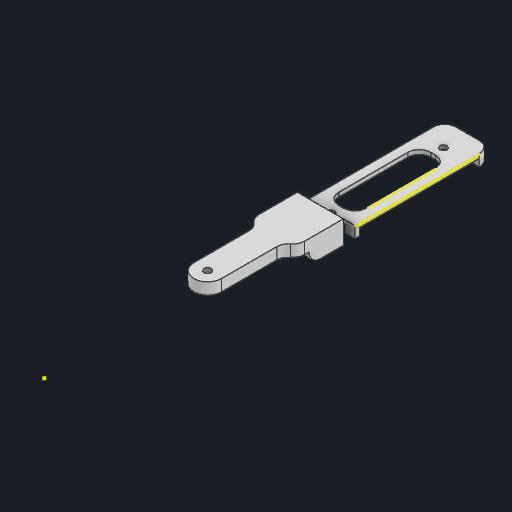
# Autodesk Inventor part: SideSensor
Saved by Autodesk Inventor 2022 (Build 260153000, 153)
## iProperties
Created: 2021-10-25
Part Number: SideSensor
Material: 一般
Document SubType Name: Modeling
Designer: shiok
Density: 1 g/cm^3
Appearance: 既定
Author: shiok
Autodesk Inventor part; units mm, degrees
ref_plane "YZ Plane" through (0, 0, 0) normal (1, 0, 0) x (0, 1, 0)
ref_plane "XZ Plane" through (0, 0, 0) normal (0, 1, 0) x (-1, 0, 0)
ref_plane "XY Plane" through (0, 0, 0) normal (0, 0, 1) x (1, 0, 0)
sketch "スケッチ1" plane through (0, 0, 0) normal (0, 1, 0) x (-1, 0, 0)
  line L0 (3, -32.5) -> (-3, -32.5)
  line L1 (-3, -32.5) -> (-3, -89.5)
  line L2 (3, -89.5) -> (3, -32.5)
  line L3 (-3, -89.5) -> (0, -89.5)
  line L4 (0, -89.5) -> (3, -89.5)
  point P0 (0, 0)
  point P1 (0, -35)
  point P2 (0, -40)
  point P3 (0, -50)
  dimension "d1" = 32.5
  dimension "d2" = 2.5
  dimension "d3" = 5
  dimension "d4" = 10
  dimension "d5" = 6
  dimension "d6" = 89.5
  constraints: 10 end point, 4 vertical alignment, 2 collinear, 2 horizontal, 1 parallel, 1 perpendicular
  measures "d1" distance from line of L0 point (0, 0)
  measures "d2" distance from line of L0 point (0, -35)
  measures "d3" distance of point (0, -40) point (0, -35)
  measures "d4" distance of point (0, -50) point (0, -40)
  measures "d5" distance of L0.start L0.end
  measures "d6" distance from line of point (0, 0) L4
extrude "押し出し1" add sketch "スケッチ1" along normal blind 2.5
sketch "スケッチ2" plane through (0, 2.5, 0) normal (0, 1, 0) x (1, 0, 0)
  line L0 (-3, 32.5) -> (3, 32.5) projected
  line L1 (0, 32.5) -> (0, 35) construction
  point P0 (0, 0)
  point P1 (0, 40)
  point P2 (0, 50)
  dimension "d9" = 2.5
  dimension "d10" = 5
  dimension "d11" = 10
  constraints: 2 end point, 2 vertical alignment, 1 midpoint, 1 vertical
  measures "d9" distance from line of L0 L1.end
  measures "d10" distance of point (0, 40) L1.end
  measures "d11" distance of point (0, 50) point (0, 40)
hole "穴1" at (0, 2.5, -50) at (0, 2.5, -40) at (0, 2.5, -35) direction (0, -1, 0) diameter 1.567 depth 2.5 thread size "M2x0.4" class "6H" standard "ISO Metric profile"
sketch "スケッチ3" plane through (0, 2.5, 0) normal (0, 1, 0) x (1, 0, 0)
  line L0 (-5, 50) -> (-5, 89.5)
  line L1 (-5, 89.5) -> (5, 89.5)
  line L2 (5, 89.5) -> (5, 50)
  circle A0 centre (0, 50) radius 0.7835 projected
  line L3 (3, 89.5) -> (-3, 89.5) projected
  line L4 (5, 50) -> (0, 50)
  line L5 (0, 50) -> (-5, 50)
  point P0 (0, 0)
  point P1 (0.5, 89.5)
  point P2 (-0.5, 89.5)
  point P3 (-0.7835, 50)
  point P4 (0.7835, 50)
  dimension "d22" = 10
  constraints: 10 end point, 2 collinear, 2 equal length, 1 horizontal, 1 vertical
  measures "d22" distance between parallel lines of L2 L0
extrude "押し出し2" add sketch "スケッチ3" against normal up to surface (2.5 mm away) contours L0 L1 L2 L4 A0 L5
fillet "フィレット3" radius 2.5 6 edges at (5, 1.25, -50) (3, 1.25, -50) (-5, 1.25, -50) (-3, 1.25, -50) (5, 1.25, -89.5) (-5, 1.25, -89.5)
sketch "スケッチ4" plane through (0, 0, 0) normal (0, -1, 0) x (1, 0, 0)
  line L0 (-2.5, -89.5) -> (2.5, -89.5) projected
  line L1 (2.5, -89.5) -> (-2.5, -89.5) construction
  line L2 (0, -89.5) -> (0, -86.75) construction
  line L3 (0, -86.75) -> (0, -62.25) construction
  circle A0 centre (0, -50) radius 0.7835 projected
  point P0 (0, 0)
  point P1 (0, -74.5)
  dimension "d36" = 12.25
  dimension "d42" = 24.5
  constraints: 4 end point, 2 coincident, 2 midpoint, 1 point on line, 1 vertical
  measures "d36" distance of L3.end A0.centre
  measures "d42" distance of point (0, -86.75) point (0, -62.25)
hole "穴2" at (0, 0, -86.75) at (0, 0, -62.25) direction (0, 1, 0) diameter 1.567 depth 2.5 thread size "M2x0.4" class "6H" standard "ISO Metric profile"
sketch "スケッチ5" plane through (0, 0, 0) normal (0, -1, 0) x (1, 0, 0)
  line L0 (-2.5, -89.5) -> (2.5, -89.5) projected
  line L1 (2.5, -89.5) -> (-2.5, -89.5) construction
  line L2 (0.5, -64.5) -> (-0.5, -64.5)
  line L3 (-3, -67) -> (-3, -82)
  line L4 (-0.5, -84.5) -> (0.5, -84.5)
  line L5 (3, -82) -> (3, -67)
  line L6 (3, -64.5) -> (-3, -84.5) construction
  line L7 (3, -84.5) -> (-3, -64.5) construction
  circle A0 centre (0, -62.25) radius 0.7835 construction
  circle A1 centre (0, -86.75) radius 0.7835 construction
  line L8 (0, -62.25) -> (0, -86.75) construction
  arc A2 (3, -67) -> (0.5, -64.5) centre (0.5, -67) ccw
  arc A3 (0.5, -84.5) -> (3, -82) centre (0.5, -82) ccw
  arc A4 (-3, -82) -> (-0.5, -84.5) centre (-0.5, -82) ccw
  arc A5 (-0.5, -64.5) -> (-3, -67) centre (-0.5, -67) ccw
  point P0 (0, 0)
  point P1 (0, -74.5)
  dimension "d37" = 20
  dimension "d38" = 6
  dimension "d39" = 2.5
  constraints: 14 end point, 8 point on circle, 8 point on line, 8 tangent, 4 centre point, 3 equal radius, 3 midpoint, 2 parallel, 1 horizontal, 1 perpendicular, 1 vertical
  measures "d37" distance of L7.end L6.end
  measures "d38" distance of L6.end L7.start
  measures "d39" radius of A2
extrude "押し出し3" cut sketch "スケッチ5" against normal up to surface (2.5 mm away)
sketch "スケッチ6" plane through (0, 2.5, 0) normal (0, 1, 0) x (1, 0, 0)
  circle A0 centre (0, 40) radius 0.7835 projected
  circle A1 centre (0, 35) radius 0.7835 projected
  point P0 (0, 0)
extrude "押し出し4" add sketch "スケッチ6" against normal up to surface (2.5 mm away)
fillet "フィレット4" radius 3 2 edges at (3, 1.25, -32.5) (-3, 1.25, -32.5)
sketch "スケッチ8" plane through (0, 2.5, 0) normal (0, 1, 0) x (1, 0, 0)
  circle A0 centre (0, 50) radius 0.7835 projected
  point P0 (0, 0)
extrude "押し出し5" add sketch "スケッチ8" against normal up to surface (2.5 mm away)
sketch "スケッチ9" plane through (0, 0, 0) normal (0, -1, 0) x (1, 0, 0)
  arc A0 (3, -35.5) -> (-3, -35.5) centre (0, -35.5) ccw projected
  line L0 (-3, -47.5505) -> (-3, -35.5) projected
  arc A1 (-4, -49.5505) -> (-3, -47.5505) centre (-5.5, -47.5505) ccw projected
  arc A2 (-4, -49.5505) -> (-5, -51.5505) centre (-2.5, -51.5505) ccw projected
  line L1 (-5, -51.5505) -> (-5, -87) projected
  arc A3 (-5, -87) -> (-2.5, -89.5) centre (-2.5, -87) ccw projected
  line L2 (-2.5, -89.5) -> (2.5, -89.5) projected
  arc A4 (2.5, -89.5) -> (5, -87) centre (2.5, -87) ccw projected
  line L3 (5, -87) -> (5, -51.5505) projected
  arc A5 (5, -51.5505) -> (4, -49.5505) centre (2.5, -51.5505) ccw projected
  arc A6 (3, -47.5505) -> (4, -49.5505) centre (5.5, -47.5505) ccw projected
  line L4 (3, -35.5) -> (3, -47.5505) projected
  line L5 (3, -67) -> (3, -82) projected
  arc A7 (0.5, -84.5) -> (3, -82) centre (0.5, -82) ccw projected
  line L6 (0.5, -84.5) -> (-0.5, -84.5) projected
  arc A8 (-3, -82) -> (-0.5, -84.5) centre (-0.5, -82) ccw projected
  line L7 (-3, -82) -> (-3, -67) projected
  arc A9 (-0.5, -64.5) -> (-3, -67) centre (-0.5, -67) ccw projected
  line L8 (-0.5, -64.5) -> (0.5, -64.5) projected
  arc A10 (3, -67) -> (0.5, -64.5) centre (0.5, -67) ccw projected
  circle A11 centre (0, -86.75) radius 0.7835 projected
  circle A12 centre (0, -62.25) radius 0.7835 projected
  line L9 (-5, -51.5505) -> (-5, -87) projected
  line L10 (5, -89.5) -> (-5, -89.5)
  line L11 (-5, -89.5) -> (-5, -59.5)
  line L12 (-5, -59.5) -> (5, -59.5)
  line L13 (5, -59.5) -> (5, -89.5)
  line L14 (5, -87) -> (5, -51.5505) projected
  line L15 (-2.5, -89.5) -> (2.5, -89.5) projected
  line L16 (5, -59.5) -> (3, -59.5)
  line L17 (3, -59.5) -> (3, -63.5)
  line L18 (3, -63.5) -> (5, -63.5)
  line L19 (5, -63.5) -> (5, -59.5)
  line L20 (0, -35.5) -> (0, -86.75)
  line L21 (-3, -59.5) -> (-3, -63.5)
  line L22 (-3, -63.5) -> (-5, -63.5)
  point P0 (0, 0)
  dimension "d56" = 30
  dimension "d67" = 2
  dimension "d68" = 4
  constraints: 22 end point, 4 parallel, 3 symmetric about line, 2 collinear, 2 horizontal, 2 perpendicular, 1 point on line, 1 vertical
  measures "d56" distance of L10.end L11.end
  measures "d67" distance of L18.end L17.end
  measures "d68" distance of L17.end L16.end
extrude "押し出し6" cut sketch "スケッチ9" against normal blind 1.6 contours L3 A4 L2 A3 L1 L22 L21 L12 L17 L18
sketch "スケッチ10" plane through (0, 2.5, 0) normal (0, 1, 0) x (1, 0, 0)
  arc A0 (-2.5, 89.5) -> (-5, 87) centre (-2.5, 87) ccw projected
  line L0 (-5, 87) -> (5, 87)
  line L1 (5, 87) -> (5, 92)
  line L2 (5, 92) -> (-5, 92)
  line L3 (-5, 92) -> (-5, 87)
  circle A1 centre (0, 86.75) radius 0.7835 projected
  point P0 (0, 0)
  point P1 (-0.7425, 87)
  point P2 (0.7425, 87)
  dimension "d59" = 10
  dimension "d60" = 5
  constraints: 8 end point, 2 parallel, 1 horizontal, 1 perpendicular
  measures "d59" distance of L2.end L1.end
  measures "d60" distance of L1.end L0.end
extrude "押し出し7" add sketch "スケッチ10" against normal up to surface (0.9 mm away) contours L3 L2 L1 L0 A1
sketch "スケッチ11" plane through (0, 1.6, 0) normal (0, -1, 0) x (1, 0, 0)
  line L0 (5, -63.5) -> (5, -92) projected
  line L1 (-5, -92) -> (-5, -51.5505) projected
  line L2 (5, -89.5) -> (-5, -89.5)
  line L3 (-5, -89.5) -> (-5, -92)
  line L4 (-5, -92) -> (5, -92)
  line L5 (5, -92) -> (5, -89.5)
  line L6 (5, -92) -> (-5, -92) projected
  point P0 (0, 0)
  point P1 (5, -59.5)
  dimension "d63" = 2.5
  constraints: 8 end point, 2 parallel, 2 point on line, 1 collinear, 1 horizontal, 1 perpendicular
  measures "d63" distance between parallel lines of L4 L2
extrude "押し出し8" add sketch "スケッチ11" along normal up to surface (1.6 mm away)
fillet "フィレット5" radius 2.5 2 edges at (5, 1.25, -92) (-5, 1.25, -92)
sketch "スケッチ12" plane through (0, 2.5, 0) normal (0, 1, 0) x (1, 0, 0)
  line L0 (5, 32.5) -> (-5, 32.5)
  line L1 (-5, 32.5) -> (-5, 57.5)
  line L2 (-5, 57.5) -> (5, 57.5)
  line L3 (5, 57.5) -> (5, 32.5)
  line L4 (5, 51.5505) -> (5, 89.5) projected
  arc A0 (-3, 35.5) -> (3, 35.5) centre (0, 35.5) ccw projected
  arc A1 (-2.5, 92) -> (-5, 89.5) centre (-2.5, 89.5) ccw projected
  line L5 (-5, 89.5) -> (-5, 51.5505) projected
  arc A2 (-5, 51.5505) -> (-4, 49.5505) centre (-2.5, 51.5505) ccw projected
  arc A3 (-3, 47.5505) -> (-4, 49.5505) centre (-5.5, 47.5505) ccw projected
  line L6 (-3, 47.5505) -> (-3, 35.5) projected
  arc A4 (-3, 35.5) -> (3, 35.5) centre (0, 35.5) ccw projected
  line L7 (3, 35.5) -> (3, 47.5505) projected
  arc A5 (4, 49.5505) -> (3, 47.5505) centre (5.5, 47.5505) ccw projected
  arc A6 (4, 49.5505) -> (5, 51.5505) centre (2.5, 51.5505) ccw projected
  line L8 (5, 51.5505) -> (5, 89.5) projected
  arc A7 (5, 89.5) -> (2.5, 92) centre (2.5, 89.5) ccw projected
  line L9 (2.5, 92) -> (-2.5, 92) projected
  circle A8 centre (0, 86.75) radius 0.7835 projected
  circle A9 centre (0, 62.25) radius 0.7835 projected
  line L10 (3, 82) -> (3, 67) projected
  arc A10 (0.5, 64.5) -> (3, 67) centre (0.5, 67) ccw projected
  line L11 (0.5, 64.5) -> (-0.5, 64.5) projected
  arc A11 (-3, 67) -> (-0.5, 64.5) centre (-0.5, 67) ccw projected
  line L12 (-3, 67) -> (-3, 82) projected
  arc A12 (-0.5, 84.5) -> (-3, 82) centre (-0.5, 82) ccw projected
  line L13 (-0.5, 84.5) -> (0.5, 84.5) projected
  arc A13 (3, 82) -> (0.5, 84.5) centre (0.5, 82) ccw projected
  point P0 (0, 0)
  point P1 (-3, 35.5)
  dimension "d69" = 10
  dimension "d70" = 25
  constraints: 8 end point, 2 parallel, 1 collinear, 1 horizontal, 1 perpendicular, 1 tangent
  measures "d69" distance of L1.end L2.end
  measures "d70" distance of L0.end L1.end
extrude "押し出し9" add sketch "スケッチ12" along normal blind 2.5 contours A0 L6 A3 A2 L1 L2 L3 A6 A5 L7
sketch "スケッチ13" plane through (0, 5, 0) normal (0, 1, 0) x (1, 0, 0)
  arc A0 (-3, 35.5) -> (3, 35.5) centre (0, 35.5) ccw projected
  line L0 (3, 35.5) -> (3, 47.5505) projected
  arc A1 (4, 49.5505) -> (3, 47.5505) centre (5.5, 47.5505) ccw projected
  arc A2 (4, 49.5505) -> (5, 51.5505) centre (2.5, 51.5505) ccw projected
  line L1 (5, 51.5505) -> (5, 57.5) projected
  line L2 (5, 57.5) -> (-5, 57.5) projected
  line L3 (-5, 57.5) -> (-5, 51.5505) projected
  arc A3 (-5, 51.5505) -> (-4, 49.5505) centre (-2.5, 51.5505) ccw projected
  arc A4 (-3, 47.5505) -> (-4, 49.5505) centre (-5.5, 47.5505) ccw projected
  line L4 (-3, 47.5505) -> (-3, 35.5) projected
  point P0 (0, 0)
extrude "押し出し10" cut sketch "スケッチ13" along normal blind 2.5 from surface at -5
sketch "スケッチ15" plane through (-5, 0, -57.5) normal (0, 0, 1) x (1, 0, 0)
  line L0 (10, 0) -> (0, 0) projected
  line L1 (10, 2.5) -> (10, 0) projected
  line L2 (0, 2.5) -> (10, 2.5) projected
  line L3 (0, 0) -> (0, 2.5) projected
  point P0 (5, 0)
extrude "押し出し11" add sketch "スケッチ15" along normal blind 5
sketch "スケッチ16" plane through (5, 2.5, -57.5) normal (0, 0, -1) x (-1, 0, 0)
  line L0 (10, 0) -> (0, 0) projected
  line L1 (10, 0) -> (10, 2.5) projected
  line L2 (0, 2.5) -> (10, 2.5) projected
  line L3 (0, 0) -> (0, 2.5) projected
  point P0 (5, -2.5)
extrude "押し出し12" add sketch "スケッチ16" along normal blind 5
fillet "フィレット6" [suppressed]
fillet "フィレット7" radius 2.5 1 edges at (0, 0, -52.5)
sketch "スケッチ17" plane through (0, 5, 0) normal (0, 1, 0) x (1, 0, 0)
  arc A0 (-3, 35.5) -> (3, 35.5) centre (0, 35.5) ccw projected
  line L0 (3, 35.5) -> (3, 47.5505) projected
  arc A1 (4, 49.5505) -> (3, 47.5505) centre (5.5, 47.5505) ccw projected
  arc A2 (4, 49.5505) -> (5, 51.5505) centre (2.5, 51.5505) ccw projected
  line L1 (5, 51.5505) -> (5, 62.5) projected
  line L2 (-5, 62.5) -> (5, 62.5) projected
  line L3 (-5, 51.5505) -> (-5, 62.5) projected
  arc A3 (-5, 51.5505) -> (-4, 49.5505) centre (-2.5, 51.5505) ccw projected
  arc A4 (-3, 47.5505) -> (-4, 49.5505) centre (-5.5, 47.5505) ccw projected
  line L4 (-3, 47.5505) -> (-3, 35.5) projected
  line L5 (-5, 60) -> (-5, 57.5) projected
  line L6 (-5, 57.5) -> (5, 57.5) projected
  line L7 (5, 57.5) -> (5, 60) projected
  line L8 (5, 60) -> (-5, 60) projected
  line L9 (3, 59.5) -> (3, 63.5) projected
  line L10 (5, 62.5) -> (5, 89.5) projected
  arc A5 (5, 89.5) -> (2.5, 92) centre (2.5, 89.5) ccw projected
  line L11 (2.5, 92) -> (-2.5, 92) projected
  arc A6 (-2.5, 92) -> (-5, 89.5) centre (-2.5, 89.5) ccw projected
  line L12 (-5, 89.5) -> (-5, 62.5) projected
  circle A7 centre (0, 86.75) radius 0.7835 projected
  line L13 (3, 82) -> (3, 67) projected
  arc A8 (0.5, 64.5) -> (3, 67) centre (0.5, 67) ccw projected
  line L14 (0.5, 64.5) -> (-0.5, 64.5) projected
  arc A9 (-3, 67) -> (-0.5, 64.5) centre (-0.5, 67) ccw projected
  line L15 (-3, 67) -> (-3, 82) projected
  arc A10 (-0.5, 84.5) -> (-3, 82) centre (-0.5, 82) ccw projected
  line L16 (-0.5, 84.5) -> (0.5, 84.5) projected
  arc A11 (3, 82) -> (0.5, 84.5) centre (0.5, 82) ccw projected
  arc A12 (0.7425, 62.5) -> (-0.7425, 62.5) centre (0, 62.25) ccw projected
  line L17 (0.7425, 62.5) -> (5, 62.5) projected
  line L18 (-5, 62.5) -> (-0.7425, 62.5) projected
  point P0 (0, 0)
extrude "押し出し13" cut sketch "スケッチ17" against normal blind 5 contours L4 A4 A3 L3 L6 L1 A2 A1 L0 A0 | L3 L8 L1 L6 | L12 A6 L11 A5 L10 L2 A12 | A7 keep common part
fillet "フィレット8" [suppressed]
sketch "スケッチ18" plane through (0, 5, 0) normal (0, 1, 0) x (1, 0, 0)
  arc A0 (-3, 35.5) -> (3, 35.5) centre (0, 35.5) ccw projected
  point P0 (0, 0)
  constraints: 1 coincident
hole "穴4" at (0, 5, -35.5) direction (0, -1, 0) diameter 1.567 depth 6.3 thread size "M2x0.4" class "6H" standard "ISO Metric profile"
sketch "スケッチ19" plane through (0, 2.5, 0) normal (0, 1, 0) x (1, 0, 0)
  point P0 (0, 0)
sketch "スケッチ20" plane through (0, 2.5, 0) normal (0, 1, 0) x (1, 0, 0)
  line L0 (3, 82) -> (3, 67) projected
  line L1 (5, 62.5) -> (5, 89.5) projected
  point P0 (0, 0)
equation "\"d17\" = d11"
